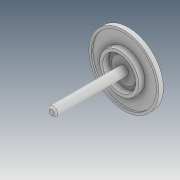
# Autodesk Inventor part: PMSeal
Saved by Autodesk Inventor 2020 (Build 240168000, 168)
## iProperties
Created: 2020-05-07
Part Number: PMSeal
Material: Generic
Document SubType Name: Modeling
Designer: Theo Cominotto
Density: 1 g/cm^3
Appearance: Default
Author: Theo Cominotto
Autodesk Inventor part; units mm, degrees
ref_plane "YZ Plane" through (0, 0, 0) normal (1, 0, 0) x (0, 1, 0)
ref_plane "XZ Plane" through (0, 0, 0) normal (0, 1, 0) x (-1, 0, 0)
ref_plane "XY Plane" through (0, 0, 0) normal (0, 0, 1) x (1, 0, 0)
sketch "Sketch1" plane through (0, 0, 0) normal (0, 0, 1) x (1, 0, 0)
  circle A0 centre (0, 0) radius 11.4
  dimension "d0" = 22.8
  constraints: 1 centre point, 1 coincident
  measures "d0" diameter of A0
extrude "Extrusion1" add sketch "Sketch1" along normal blind 1
sketch "Sketch2" plane through (0, 0, 1) normal (0, 0, 1) x (1, 0, 0)
  circle A0 centre (0, 0) radius 11.4 projected
  circle A1 centre (0, 0) radius 10.6
  dimension "d3" = 0.8
  constraints: 1 centre point
  measures "d3" radial gap between concentric circles of A0 A1
extrude "Extrusion2" add sketch "Sketch2" along normal blind 0.5
sketch "Sketch3" plane through (0, 0, 1) normal (0, 0, 1) x (1, 0, 0)
  circle A0 centre (0, 0) radius 6.375
  circle A1 centre (0, 0) radius 5.375
  dimension "d6" = 12.75
  dimension "d7" = 10.75
  constraints: 2 centre point, 2 coincident
  measures "d6" diameter of A0
  measures "d7" diameter of A1
extrude "Extrusion3" add sketch "Sketch3" along normal blind 2
sketch "Sketch4" plane through (0, 0, 1) normal (0, 0, 1) x (1, 0, 0)
  circle A0 centre (0, 0) radius 1.425
  dimension "d10" = 2.85
  constraints: 1 centre point, 1 coincident
  measures "d10" diameter of A0
extrude "Extrusion4" add sketch "Sketch4" along normal blind 24.1
fillet "Fillet1" radius 0.6 1 edges at (-1.425, 0, 25.1)
sketch "Sketch5" plane through (0, 0, 1) normal (0, 0, 1) x (1, 0, 0)
  circle A0 centre (0, 0) radius 4.125
  dimension "d14" = 8.25
  constraints: 1 centre point, 1 coincident
  measures "d14" diameter of A0
extrude "Extrusion5" add sketch "Sketch5" along normal blind 0.4
body "Solid1"
